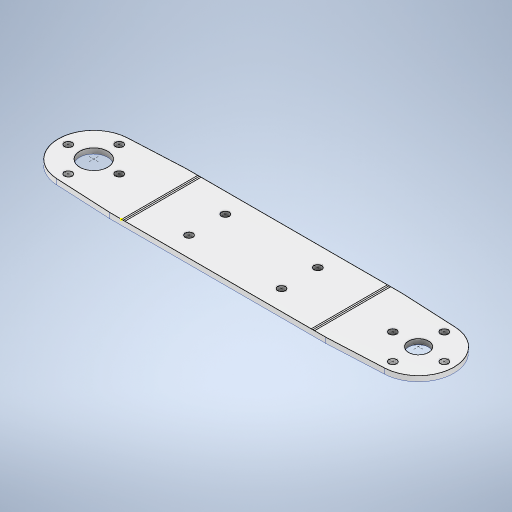
# Autodesk Inventor part: CAM_ㄷ_frame_2
Saved by Autodesk Inventor 2023 (Build 270158000, 158)
## iProperties
Created: 2022-10-27
Part Number: CAM_ㄷ_frame_2
Material: Aluminum 6061
Document SubType Name: Sheet Metal
Designer: chanh
Density: 2.7 g/cm^3
Sheet Metal Rule: Default_mm
Appearance: Aluminum - Flat
Author: chanh
Autodesk Inventor part; units mm, degrees
ref_plane "YZ Plane" through (0, 0, 0) normal (1, 0, 0) x (0, 1, 0)
ref_plane "XZ Plane" through (0, 0, 0) normal (0, 1, 0) x (-1, 0, 0)
ref_plane "XY Plane" through (0, 0, 0) normal (0, 0, 1) x (1, 0, 0)
sketch "Sketch2" plane through (0, 0, 0) normal (0, 1, 0) x (-1, 0, 0)
  line L0 (-0.4496, -21) -> (-0.4496, 0)
  line L1 (-52.7289, -21) -> (-52.7289, 0)
  circle A0 centre (-13.0893, -5.5) radius 1.05
  circle A1 centre (-38.5893, -5.5) radius 1.05
  circle A2 centre (-38.5893, -15.5) radius 1.05
  circle A3 centre (-13.0893, -15.5) radius 1.05
  circle A4 centre (11.165, -10.5) radius 1.05
  circle A5 centre (25.215, -10.5) radius 1.05
  circle A6 centre (18.19, -3.475) radius 1.05
  circle A7 centre (18.19, -17.525) radius 1.05
  circle A8 centre (18.19, -10.5) radius 3.85
  circle A9 centre (-71.3686, -10.5) radius 2.75
  circle A10 centre (-78.4686, -10.5) radius 1.05
  circle A11 centre (-71.3686, -3.4) radius 1.05
  circle A12 centre (-64.2686, -10.5) radius 1.05
  circle A13 centre (-71.3686, -17.6) radius 1.05
  arc A14 (18.6693, -20.2382) -> (18.6693, -0.7618) centre (18.19, -10.5) ccw
  line L2 (3.19, -21) -> (18.6693, -20.2382)
  line L3 (18.6693, -0.7618) -> (3.19, 0)
  line L4 (-56.3686, 0) -> (3.19, 0)
  line L5 (3.19, -21) -> (-56.3686, -21)
  line L6 (-71.8478, -0.7618) -> (-56.3686, 0)
  arc A15 (-71.8478, -0.7618) -> (-71.8478, -20.2382) centre (-71.3686, -10.5) ccw
  line L7 (-56.3686, -21) -> (-71.8478, -20.2382)
  line L8 (-53.1786, -21) -> (-53.1786, 0)
  line L9 (-52.2793, 0) -> (-52.2793, -21)
  line L10 (-0.8993, -21) -> (-0.8993, 0)
  line L11 (0, 0) -> (0, -21)
  constraints: 24 end point, 16 centre point, 12 equal radius, 12 point on line, 7 parallel, 6 vertical, 4 point on circle, 4 tangent, 2 horizontal, 2 perpendicular, 55 other
extrude "Plate2" add sketch "Sketch2" against normal blind 1.5
equation "\"d1\" = Thickness"
equation "\"BendReliefWidth\" = Thickness"
equation "\"BendReliefDepth\" = 0.5 * Thickness"
equation "\"CornerReliefSize\" = 4 * Thickness"
equation "\"MinimumRemnant\" = 2 * Thickness"
equation "\"TransitionRadius\" = BendRadius"
equation "\"JacobiRadiusSize\" = BendRadius"
equation "\"GapSize\" = Thickness"
equation "\"Thickness\" = 1.5"
equation "\"BendRadius\" = 0.31"
body "Solid2"
